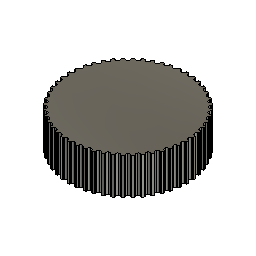
gear_52z (Autodesk Fusion 360 design; units mm, degrees)
Autodesk Fusion 360 part; units mm, degrees
sketch "Sketch1" plane through (0, 0, 0) normal (0, 0, 1) x (1, 0, 0) in component "gt2 pulley"
  circle A0 centre (0, 0) radius 16.5521 construction
  circle A1 centre (0, 0) radius 15.5481 construction
  line L0 (0, 0) -> (0, 16.5521) construction
  line L1 (0, 0) -> (0.9994, 16.5219) construction
  line L2 (0, 0) -> (1.407, 16.4922) construction
  circle A2 centre (0, 0) radius 16.2981 construction
  arc A3 (0.3887, 16.1584) -> (0.457, 15.8675) centre (1.3854, 16.2391) ccw
  circle A4 centre (0, 0) radius 16.1481 construction
  arc A5 (0.2413, 16.2963) -> (0, 16.2981) centre (0, 0) ccw
  arc A6 (0.3887, 16.1584) -> (0.2413, 16.2963) centre (0.2392, 16.1463) ccw
  arc A7 (0.457, 15.8675) -> (0.9388, 15.5197) centre (0.9723, 16.0737) ccw
  arc A8 (0, 16.2981) -> (-0.2413, 16.2963) centre (0, 0) ccw
  arc A9 (-0.2413, 16.2963) -> (-0.3887, 16.1584) centre (-0.2392, 16.1463) ccw
  arc A10 (-0.457, 15.8675) -> (-0.3887, 16.1584) centre (-1.3854, 16.2391) ccw
  arc A11 (-0.9388, 15.5197) -> (-0.457, 15.8675) centre (-0.9723, 16.0737) ccw
  arc A12 (0.9388, 15.5197) -> (-0.9388, 15.5197) centre (0, 0) ccw
  point P0 (1.3854, 16.2391)
  point P1 (0, 16.2981)
  dimension "d18" = 33.1042
  dimension "d19" = 3.462
  dimension "d22" = 1.004
  dimension "d24" = 0.75
  dimension "d26" = 1
  dimension "d27" = 0.15
  dimension "d28" = 0.15
  dimension "d47" = 0.555
  dimension "d52" = 3.812
  constraint coincident A0.centre A1.centre
  constraint coincident A0 L0.end
  constraint vertical L0
  constraint coincident A0 L1.end
  constraint coincident A0 L2.end
  constraint concentric A1 A2
  constraint coincident A1 A7.end
  constraint coincident L1 A7.end
  constraint coincident A2 P0
  constraint coincident L2 P0
  constraint coincident P0 A3.centre
  constraint coincident A2 P1
  constraint coincident L0 P1
  constraint concentric A2 A4
  constraint coincident P1 A5.end
  constraint coincident A4 A6.centre
  constraint coincident A3.start A6.start
  constraint tangent A3 A6
  constraint tangent A3 A7
  constraint symmetric L0 A7.end A11.start
  constraint symmetric L0 A3.start A9.end
  constraint symmetric L0 A3.end A10.start
  constraint symmetric L0 A3 A10
  constraint symmetric L0 A5.start A8.end
  constraint symmetric L0 P1 A5.end
  constraint symmetric L0 A5 A8
  constraint symmetric L0 A6 A9
  constraint symmetric L0 A7 A11
  constraint coincident A1 A11.start
  constraint tangent A1 A7
  constraint coincident L1 A7.centre
  measures "d18" diameter of A0
  measures "d19" angle of L0 L1
  measures "d22" distance of A0 A1
  measures "d24" distance of A1 A2
  measures "d26" radius of A3
  measures "d27" distance of A2 A4
  measures "d28" radius of A6
  measures "d47" radius of A7
extrude "Extrude1" add sketch "Sketch1" along normal blind 10 makes body 1
pattern_circular "C-Pattern1" count 52 over 360 about axis through (0, 0, 1.75) along (0, 0, 1) of bodies 1 makes body 2 at (-2.391, 15.3632, 6.6667) makes body 3 at (-3.0077, 15.2544, 3.3333) makes body 4 at (-4.8245, 14.7807, 3.3333) makes body 5 at (-7.6835, 13.5169, 6.6667) makes body 6 at (-9.2568, 12.4922, 6.6667) makes body 7 at (-10.6951, 11.2854, 6.6667) makes body 8 at (-11.9774, 9.9139, 6.6667) makes body 9 at (-12.3668, 9.4236, 3.3333) makes body 10 at (-13.7184, 7.3178, 6.6667) makes body 11 at (-14.2627, 6.1902, 3.3333) makes body 12 at (-15.2127, 3.2122, 6.6667) makes body 13 at (-15.4889, 1.3551, 6.6667) makes body 14 at (-15.5394, -0.5218, 6.6667) makes body 15 at (-15.5057, -1.147, 3.3333) makes body 16 at (-15.1209, -3.6195, 6.6667) makes body 17 at (-14.5004, -5.6109, 6.6667) makes body 18 at (-13.5169, -7.6835, 6.6667) makes body 19 at (-13.1966, -8.2215, 3.3333) makes body 20 at (-11.2854, -10.6951, 6.6667) makes body 21 at (-10.8456, -11.1408, 3.3333) makes body 22 at (-9.4236, -12.3668, 3.3333) makes body 23 at (-7.3178, -13.7184, 6.6667) makes body 24 at (-5.0225, -14.7146, 6.6667) makes body 25 at (-4.4259, -14.9049, 3.3333) makes body 26 at (-1.3551, -15.4889, 6.6667) makes body 27 at (0.5218, -15.5394, 6.6667) makes body 28 at (2.391, -15.3632, 6.6667) makes body 29 at (4.2254, -14.9629, 6.6667) makes body 30 at (5.6109, -14.5004, 6.6667) makes body 31 at (7.133, -13.8154, 6.6667) makes body 32 at (9.2568, -12.4922, 6.6667) makes body 33 at (10.6951, -11.2854, 6.6667) makes body 34 at (11.1408, -10.8456, 3.3333) makes body 35 at (13.1966, -8.2215, 6.6667) makes body 36 at (13.7184, -7.3178, 6.6667) makes body 37 at (14.2627, -6.1902, 3.3333) makes body 38 at (14.9049, -4.4259, 3.3333) makes body 39 at (15.5057, -1.147, 6.6667) makes body 40 at (15.5394, 0.5218, 6.6667) makes body 41 at (15.4218, 1.9777, 6.6667) makes body 42 at (15.1209, 3.6195, 6.6667) makes body 43 at (14.5004, 5.6109, 6.6667) makes body 44 at (13.4126, 7.8643, 6.6667) makes body 45 at (12.8548, 8.7462, 6.6667) makes body 46 at (11.2854, 10.6951, 6.6667) makes body 47 at (10.8456, 11.1408, 3.3333) makes body 48 at (8.398, 13.085, 6.6667) makes body 49 at (7.3178, 13.7184, 6.6667) makes body 50 at (5.6109, 14.5004, 6.6667) makes body 51 at (4.4259, 14.9049, 3.3333) makes body 52 at (1.3551, 15.4889, 6.6667)
sketch "Sketch2" plane through (0, 0, 10) normal (0, 0, 1) x (-1, 0, 0)
  arc A0 (-7.8533, -14.127) -> (-7.787, -14.3175) centre (-7.7153, -14.1857) ccw
  arc A1 (-7.787, -14.3175) -> (-7.3596, -14.5418) centre (0, 0) ccw
  arc A2 (-7.3596, -14.5418) -> (-7.1651, -14.4882) centre (-7.2918, -14.408) ccw
  arc A3 (-6.9693, -14.2623) -> (-7.1651, -14.4882) centre (-6.32, -15.0229) ccw
  arc A4 (-6.3811, -14.1783) -> (-6.9693, -14.2623) centre (-6.6089, -14.6844) ccw
  arc A5 (-8.0436, -13.3058) -> (-6.3811, -14.1783) centre (0, 0) ccw
  arc A6 (-7.7787, -13.8375) -> (-8.0436, -13.3058) centre (-8.3307, -13.7807) ccw
  arc A7 (-7.8533, -14.127) -> (-7.7787, -13.8375) centre (-8.7734, -13.7352) ccw
  circle A8 centre (0, 0) radius 15.5481
  constraint concentric A1 A8
extrude "Extrude2" add sketch "Sketch2" against normal blind 10 contours A5 A8 bodies 1 2 3 4 5 6 7 8 9 10 11 12 13 14 15 16 17 18 19 20 21 22 23 24 25 26 27 28 29 30 31 32 33 34 35 36 37 38 39 40 41 42 43 44 45 46 47 48 49 50 51 52
extrude "Extrude4" [suppressed] in component "gt2 pulley"
pattern_circular "C-Pattern7" [suppressed] in component "gt2 pulley"
extrude "Extrude3" [suppressed] in component "gt2 pulley"
pattern_circular "C-Pattern6" [suppressed] in component "gt2 pulley"
extrude "Extrude2'" [suppressed] in component "gt2 pulley"
pattern_circular "C-Pattern5" [suppressed] in component "gt2 pulley"
extrude "Extrude1'" [suppressed] in component "gt2 pulley"
pattern_circular "C-Pattern4" [suppressed] in component "gt2 pulley"
pattern_circular "C-Pattern3" [suppressed] in component "gt2 pulley"
pattern_circular "C-Pattern2" [suppressed] in component "gt2 pulley"
pattern_circular "C-Pattern1'" [suppressed] in component "gt2 pulley"
copy_body "Body->Comp1" [suppressed] in component "Component"
copy_body "Body->Comp2" [suppressed] in component "Component'"
copy_body "Body->Comp3" [suppressed] in component "Component''"
copy_body "Body->Comp4" [suppressed] in component "Component'''"
copy_body "Body->Comp5" [suppressed] in component "Component''''"
copy_body "Body->Comp6" [suppressed] in component "Component'''''"
copy_body "Body->Comp7" [suppressed] in component "Component''''''"
copy_body "Body->Comp8" [suppressed] in component "Component'''''''"
copy_body "Body->Comp9" [suppressed] in component "Component''''''''"
copy_body "Body->Comp10" [suppressed] in component "Component'''''''''"
copy_body "Body->Comp11" [suppressed] in component "Component''''''''''"
copy_body "Body->Comp12" [suppressed] in component "Component'''''''''''"
copy_body "Body->Comp13" [suppressed] in component "Component''''''''''''"
copy_body "Body->Comp14" [suppressed] in component "Component'''''''''''''"
copy_body "Body->Comp15" [suppressed] in component "Component''''''''''''''"
copy_body "Body->Comp16" [suppressed] in component "Component'''''''''''''''"
copy_body "Body->Comp17" [suppressed] in component "Component''''''''''''''''"
copy_body "Body->Comp18" [suppressed] in component "Component'''''''''''''''''"
copy_body "Body->Comp19" [suppressed] in component "Component''''''''''''''''''"
copy_body "Body->Comp20" [suppressed] in component "Component'''''''''''''''''''"
component "gt2 pulley" placed x (1, 0, 0) y (0, 1, 0) z (0, 0, 1) at (0, 0, 0)
equation "NumTeeth = 52" comment "min 20"
equation "ToothPitch = 2 mm"
equation "PullyDia = NumTeeth * ToothPitch / PI"
equation "ToothAng = ( ( 360 / NumTeeth ) * 1 deg )"
equation "TransOffsetAngle = ToothAng * 0.2"
equation "Sholulder_Radius = 0.15 mm"
equation "Root_Radius = 0.555 mm"
equation "TransRadius = 1 mm"
equation "ToolHeight = 0.75 mm"
equation "PLD = 0.254 mm"
equation "d18 = PullyDia"
equation "d19 = ToothAng / 2"
equation "d22 = PLD + ToolHeight"
equation "d24 = ToolHeight"
equation "d26 = TransRadius"
equation "d27 = Sholulder_Radius"
equation "d31 = NumTeeth"
equation "d33 = NumTeeth"
equation "d35 = NumTeeth"
equation "d37 = NumTeeth"
equation "d41 = NumTeeth"
equation "d45 = NumTeeth"
equation "d47 = Root_Radius"
equation "d50 = NumTeeth"
